Autodesk Inventor part; units mm, degrees
(part 2 of 2)
  line L320 (-28.6263, 16.0044) -> (-25.6449, 16.0044)
  line L321 (-25.6449, 18.3241) -> (-28.6263, 18.3241)
  line L322 (-29.7503, 19.4482) -> (-24.5209, 19.4482)
  line L323 (-29.5884, 13.8513) -> (-27.9357, 13.8513)
  line L324 (-29.5884, 12.8808) -> (-29.5884, 13.8513)
  line L325 (-29.7503, 14.8804) -> (-29.7503, 19.4482)
  line L326 (-26.6942, 13.8513) -> (-19.7097, 13.8513)
  line L327 (-23.8, 11.9101) -> (-23.8, 12.8808)
  line L328 (-25.8364, 11.9101) -> (-23.8, 11.9101)
  line L329 (-24.7124, 10.786) -> (-24.7124, 8.4664)
  line L330 (-21.731, 8.4664) -> (-21.731, 10.786)
  line L331 (-24.7124, 8.4664) -> (-21.731, 8.4664)
  line L332 (-21.731, 10.786) -> (-24.7124, 10.786)
  line L333 (-26.6942, 14.8804) -> (-26.6942, 13.8513)
  line L334 (-24.5209, 14.8804) -> (-26.6942, 14.8804)
  line L335 (-20.607, 11.9101) -> (-20.607, 7.3423)
  line L336 (-20.607, 7.3423) -> (-25.8364, 7.3423)
  line L337 (-25.8364, 7.3423) -> (-25.8364, 11.9101)
  line L338 (-27.9357, 14.8804) -> (-29.7503, 14.8804)
  line L339 (-45.1642, 41.8791) -> (-45.1642, 39.5595)
  line L340 (-49.1744, 38.4046) -> (-54.4039, 38.4046)
  line L341 (-53.2798, 39.5287) -> (-50.2985, 39.5287)
  line L342 (-50.2985, 39.5287) -> (-50.2985, 41.8484)
  line L343 (-47.0091, 45.0028) -> (-41.2208, 45.0028)
  line L344 (-51.0994, 42.9724) -> (-49.1744, 42.9724)
  line L345 (-50.2985, 41.8484) -> (-53.2798, 41.8484)
  line L346 (-55.1231, 45.0028) -> (-48.187, 45.0028)
  line L347 (-51.0994, 44.0323) -> (-51.0994, 42.9724)
  line L348 (-52.1825, 42.9724) -> (-52.1825, 44.0323)
  line L349 (-54.4039, 42.9724) -> (-52.1825, 42.9724)
  line L350 (-52.1825, 44.0323) -> (-55.1231, 44.0323)
  line L351 (-53.2798, 41.8484) -> (-53.2798, 39.5287)
  line L352 (-54.4039, 38.4046) -> (-54.4039, 42.9724)
  line L353 (-42.8734, 44.0323) -> (-42.8734, 43.0032)
  line L354 (-48.187, 45.0028) -> (-48.187, 45.9735)
  line L355 (-49.1744, 42.9724) -> (-49.1744, 38.4046)
  line L356 (-48.187, 45.9735) -> (-50.2022, 45.9735)
  line L357 (-55.1231, 44.0323) -> (-55.1231, 45.0028)
  line L358 (-46.2882, 38.4354) -> (-46.2882, 43.0032)
  line L359 (-42.1828, 39.5595) -> (-42.1828, 41.8791)
  line L360 (-42.1828, 41.8791) -> (-45.1642, 41.8791)
  line L361 (-45.1642, 39.5595) -> (-42.1828, 39.5595)
  line L362 (-41.0588, 38.4354) -> (-46.2882, 38.4354)
  line L363 (-41.2208, 44.0323) -> (-42.8734, 44.0323)
  line L364 (-41.2208, 45.0028) -> (-41.2208, 44.0323)
  line L365 (-41.0588, 43.0032) -> (-41.0588, 38.4354)
  line L366 (-44.1149, 44.0323) -> (-51.0994, 44.0323)
  line L367 (-47.0091, 45.9735) -> (-47.0091, 45.0028)
  line L368 (-44.9727, 45.9735) -> (-47.0091, 45.9735)
  line L369 (-46.0968, 47.0975) -> (-46.0968, 49.4172)
  line L370 (-49.0781, 49.4172) -> (-49.0781, 47.0975)
  line L371 (-46.0968, 49.4172) -> (-49.0781, 49.4172)
  line L372 (-49.0781, 47.0975) -> (-46.0968, 47.0975)
  line L373 (-44.1149, 43.0032) -> (-44.1149, 44.0323)
  line L374 (-46.2882, 43.0032) -> (-44.1149, 43.0032)
  line L375 (-50.2022, 45.9735) -> (-50.2022, 50.5413)
  line L376 (-50.2022, 50.5413) -> (-44.9727, 50.5413)
  line L377 (-44.9727, 50.5413) -> (-44.9727, 45.9735)
  line L378 (-42.8734, 43.0032) -> (-41.0588, 43.0032)
  line L379 (-29.0148, 57.3686) -> (-29.0148, 55.049)
  line L380 (-33.025, 53.8941) -> (-38.2545, 53.8941)
  line L381 (-37.1304, 55.0182) -> (-34.1491, 55.0182)
  line L382 (-34.1491, 55.0182) -> (-34.1491, 57.3379)
  line L383 (-30.8597, 60.4923) -> (-25.0713, 60.4923)
  line L384 (-34.95, 58.4619) -> (-33.025, 58.4619)
  line L385 (-34.1491, 57.3379) -> (-37.1304, 57.3379)
  line L386 (-38.9737, 60.4923) -> (-32.0376, 60.4923)
  line L387 (-34.95, 59.5218) -> (-34.95, 58.4619)
  line L388 (-36.0331, 58.4619) -> (-36.0331, 59.5218)
  line L389 (-38.2545, 58.4619) -> (-36.0331, 58.4619)
  line L390 (-36.0331, 59.5218) -> (-38.9737, 59.5218)
  line L391 (-37.1304, 57.3379) -> (-37.1304, 55.0182)
  line L392 (-38.2545, 53.8941) -> (-38.2545, 58.4619)
  line L393 (-26.724, 59.5218) -> (-26.724, 58.4927)
  line L394 (-32.0376, 60.4923) -> (-32.0376, 61.463)
  line L395 (-33.025, 58.4619) -> (-33.025, 53.8941)
  line L396 (-32.0376, 61.463) -> (-34.0527, 61.463)
  line L397 (-38.9737, 59.5218) -> (-38.9737, 60.4923)
  line L398 (-30.1388, 53.9249) -> (-30.1388, 58.4927)
  line L399 (-26.0334, 55.049) -> (-26.0334, 57.3686)
  line L400 (-26.0334, 57.3686) -> (-29.0148, 57.3686)
  line L401 (-29.0148, 55.049) -> (-26.0334, 55.049)
  line L402 (-24.9094, 53.9249) -> (-30.1388, 53.9249)
  line L403 (-25.0713, 59.5218) -> (-26.724, 59.5218)
  line L404 (-25.0713, 60.4923) -> (-25.0713, 59.5218)
  line L405 (-24.9094, 58.4927) -> (-24.9094, 53.9249)
  line L406 (-27.9655, 59.5218) -> (-34.95, 59.5218)
  line L407 (-30.8597, 61.463) -> (-30.8597, 60.4923)
  line L408 (-28.8233, 61.463) -> (-30.8597, 61.463)
  line L409 (-29.9473, 62.587) -> (-29.9473, 64.9067)
  line L410 (-32.9287, 64.9067) -> (-32.9287, 62.587)
  line L411 (-29.9473, 64.9067) -> (-32.9287, 64.9067)
  line L412 (-32.9287, 62.587) -> (-29.9473, 62.587)
  line L413 (-27.9655, 58.4927) -> (-27.9655, 59.5218)
  line L414 (-30.1388, 58.4927) -> (-27.9655, 58.4927)
  line L415 (-34.0527, 61.463) -> (-34.0527, 66.0308)
  line L416 (-34.0527, 66.0308) -> (-28.8233, 66.0308)
  line L417 (-28.8233, 66.0308) -> (-28.8233, 61.463)
  line L418 (-26.724, 58.4927) -> (-24.9094, 58.4927)
  line L419 (-32.0432, 45.0028) -> (-32.0432, 45.9735)
  line L420 (-32.0432, 45.9735) -> (-34.0584, 45.9735)
  line L421 (-27.9712, 44.0323) -> (-34.9556, 44.0323)
  line L422 (-32.9344, 47.0975) -> (-29.953, 47.0975)
  line L423 (-28.829, 45.9735) -> (-30.8654, 45.9735)
  line L424 (-32.9344, 49.4172) -> (-32.9344, 47.0975)
  line L425 (-34.0584, 45.9735) -> (-34.0584, 50.5413)
  line L426 (-29.953, 47.0975) -> (-29.953, 49.4172)
  line L427 (-29.953, 49.4172) -> (-32.9344, 49.4172)
  line L428 (-34.0584, 50.5413) -> (-28.829, 50.5413)
  line L429 (-28.829, 50.5413) -> (-28.829, 45.9735)
  line L430 (-30.8654, 45.9735) -> (-30.8654, 45.0028)
  line L431 (-33.0307, 38.4046) -> (-38.2601, 38.4046)
  line L432 (-37.1361, 39.5287) -> (-34.1547, 39.5287)
  line L433 (-34.1547, 39.5287) -> (-34.1547, 41.8484)
  line L434 (-34.9556, 42.9724) -> (-33.0307, 42.9724)
  line L435 (-34.1547, 41.8484) -> (-37.1361, 41.8484)
  line L436 (-38.9793, 45.0028) -> (-32.0432, 45.0028)
  line L437 (-36.0387, 42.9724) -> (-36.0387, 44.0323)
  line L438 (-38.9793, 44.0323) -> (-38.9793, 45.0028)
  line L439 (-36.0387, 44.0323) -> (-38.9793, 44.0323)
  line L440 (-38.2601, 42.9724) -> (-36.0387, 42.9724)
  line L441 (-37.1361, 41.8484) -> (-37.1361, 39.5287)
  line L442 (-38.2601, 38.4046) -> (-38.2601, 42.9724)
  line L443 (-34.9556, 44.0323) -> (-34.9556, 42.9724)
  line L444 (-29.0204, 41.8791) -> (-29.0204, 39.5595)
  line L445 (-30.8654, 45.0028) -> (-25.077, 45.0028)
  line L446 (-26.7296, 44.0323) -> (-26.7296, 43.0032)
  line L447 (-33.0307, 42.9724) -> (-33.0307, 38.4046)
  line L448 (-30.1445, 38.4354) -> (-30.1445, 43.0032)
  line L449 (-30.1445, 43.0032) -> (-27.9712, 43.0032)
  line L450 (-27.9712, 43.0032) -> (-27.9712, 44.0323)
  line L451 (-25.077, 45.0028) -> (-25.077, 44.0323)
  line L452 (-25.077, 44.0323) -> (-26.7296, 44.0323)
  line L453 (-26.0391, 41.8791) -> (-29.0204, 41.8791)
  line L454 (-26.7296, 43.0032) -> (-24.915, 43.0032)
  line L455 (-29.0204, 39.5595) -> (-26.0391, 39.5595)
  line L456 (-24.915, 38.4354) -> (-30.1445, 38.4354)
  line L457 (-24.915, 43.0032) -> (-24.915, 38.4354)
  line L458 (-26.0391, 39.5595) -> (-26.0391, 41.8791)
  line L459 (-15.8995, 45.0028) -> (-15.8995, 45.9735)
  line L460 (-15.8995, 45.9735) -> (-17.9146, 45.9735)
  line L461 (-11.8274, 44.0323) -> (-18.8118, 44.0323)
  line L462 (-16.7906, 47.0975) -> (-13.8092, 47.0975)
  line L463 (-12.6852, 45.9735) -> (-14.7216, 45.9735)
  line L464 (-16.7906, 49.4172) -> (-16.7906, 47.0975)
  line L465 (-17.9146, 45.9735) -> (-17.9146, 50.5413)
  line L466 (-13.8092, 47.0975) -> (-13.8092, 49.4172)
  line L467 (-13.8092, 49.4172) -> (-16.7906, 49.4172)
  line L468 (-17.9146, 50.5413) -> (-12.6852, 50.5413)
  line L469 (-12.6852, 50.5413) -> (-12.6852, 45.9735)
  line L470 (-14.7216, 45.9735) -> (-14.7216, 45.0028)
  line L471 (-16.8869, 38.4046) -> (-22.1163, 38.4046)
  line L472 (-20.9923, 39.5287) -> (-18.0109, 39.5287)
  line L473 (-18.0109, 39.5287) -> (-18.0109, 41.8484)
  line L474 (-18.8118, 42.9724) -> (-16.8869, 42.9724)
  line L475 (-18.0109, 41.8484) -> (-20.9923, 41.8484)
  line L476 (-22.8356, 45.0028) -> (-15.8995, 45.0028)
  line L477 (-19.895, 42.9724) -> (-19.895, 44.0323)
  line L478 (-22.8356, 44.0323) -> (-22.8356, 45.0028)
  line L479 (-19.895, 44.0323) -> (-22.8356, 44.0323)
  line L480 (-22.1163, 42.9724) -> (-19.895, 42.9724)
  line L481 (-20.9923, 41.8484) -> (-20.9923, 39.5287)
  line L482 (-22.1163, 38.4046) -> (-22.1163, 42.9724)
  line L483 (-18.8118, 44.0323) -> (-18.8118, 42.9724)
  line L484 (-12.8767, 41.8791) -> (-12.8767, 39.5595)
  line L485 (-14.7216, 45.0028) -> (-8.9332, 45.0028)
  line L486 (-10.5859, 44.0323) -> (-10.5859, 43.0032)
  line L487 (-16.8869, 42.9724) -> (-16.8869, 38.4046)
  line L488 (-14.0007, 38.4354) -> (-14.0007, 43.0032)
  line L489 (-14.0007, 43.0032) -> (-11.8274, 43.0032)
  line L490 (-11.8274, 43.0032) -> (-11.8274, 44.0323)
  line L491 (-8.9332, 45.0028) -> (-8.9332, 44.0323)
  line L492 (-8.9332, 44.0323) -> (-10.5859, 44.0323)
  line L493 (-9.8953, 41.8791) -> (-12.8767, 41.8791)
  line L494 (-10.5859, 43.0032) -> (-8.7712, 43.0032)
  line L495 (-12.8767, 39.5595) -> (-9.8953, 39.5595)
  line L496 (-8.7712, 38.4354) -> (-14.0007, 38.4354)
  line L497 (-8.7712, 43.0032) -> (-8.7712, 38.4354)
  line L498 (-9.8953, 39.5595) -> (-9.8953, 41.8791)
  spline S0 degree 2 poles (-57.0967, 82.1505) (-57.0967, 82.9326) (-56.5863, 84.2335) (-56.1417, 84.7028) knots 0 0 0 1 2 2 2
  spline S1 degree 2 poles (-56.1417, 84.7028) (-55.7218, 85.1557) (-54.495, 85.6579) (-53.8692, 85.6579) knots 0 0 0 1 2 2 2
  spline S2 degree 2 poles (-53.8692, 85.6579) (-53.1694, 85.6579) (-52.0332, 85.1886) (-51.6133, 84.744) knots 0 0 0 1 2 2 2
  spline S3 degree 2 poles (-51.6133, 84.744) (-51.0864, 84.1841) (-50.51, 82.3728) (-50.51, 80.9813) knots 0 0 0 1 2 2 2
  spline S4 degree 2 poles (-50.51, 80.9813) (-50.51, 79.7216) (-51.0781, 77.4657) (-51.6298, 76.7164) knots 0 0 0 1 2 2 2
  spline S5 degree 2 poles (-51.6298, 76.7164) (-52.2143, 75.926) (-53.861, 75.0945) (-55.0631, 75.0945) knots 0 0 0 1 2 2 2
  spline S6 degree 2 poles (-55.0631, 75.0945) (-55.3348, 75.0945) (-55.9523, 75.1521) (-56.2158, 75.2344) knots 0 0 0 1 2 2 2
  line L499 (-56.2158, 75.2344) -> (-56.2158, 76.5435)
  line L500 (-56.2158, 76.5435) -> (-56.1499, 76.5435)
  spline S7 degree 2 poles (-56.1499, 76.5435) (-55.977, 76.4447) (-55.2525, 76.2718) (-54.882, 76.2718) knots 0 0 0 1 2 2 2
  spline S8 degree 2 poles (-54.882, 76.2718) (-53.5481, 76.2718) (-52.025, 78.0338) (-51.9179, 79.664) knots 0 0 0 1 2 2 2
  spline S9 degree 2 poles (-51.9179, 79.664) (-52.4613, 79.2935) (-53.4493, 78.9559) (-54.0339, 78.9559) knots 0 0 0 1 2 2 2
  spline S10 degree 2 poles (-54.0339, 78.9559) (-54.5938, 78.9559) (-55.5242, 79.2029) (-55.9935, 79.557) knots 0 0 0 1 2 2 2
  spline S11 degree 2 poles (-55.9935, 79.557) (-56.5369, 79.9769) (-57.0967, 81.253) (-57.0967, 82.1505) knots 0 0 0 1 2 2 2
  spline S12 degree 2 poles (-51.885, 81.286) (-51.885, 82.3151) (-52.2637, 83.616) (-52.6013, 83.97) knots 0 0 0 1 2 2 2
  spline S13 degree 2 poles (-52.6013, 83.97) (-52.8977, 84.2994) (-53.5152, 84.5464) (-53.8775, 84.5464) knots 0 0 0 1 2 2 2
  spline S14 degree 2 poles (-53.8775, 84.5464) (-54.7173, 84.5464) (-55.7135, 83.3443) (-55.7135, 82.2081) knots 0 0 0 1 2 2 2
  spline S15 degree 2 poles (-55.7135, 82.2081) (-55.7135, 81.5659) (-55.3842, 80.7343) (-55.0219, 80.4379) knots 0 0 0 1 2 2 2
  spline S16 degree 2 poles (-55.0219, 80.4379) (-54.7585, 80.2239) (-54.108, 80.0839) (-53.7293, 80.0839) knots 0 0 0 1 2 2 2
  spline S17 degree 2 poles (-53.7293, 80.0839) (-53.2929, 80.0839) (-52.2884, 80.3885) (-51.9097, 80.6438) knots 0 0 0 1 2 2 2
  spline S18 degree 2 poles (-51.9097, 80.6438) (-51.9015, 80.7426) (-51.885, 81.0801) (-51.885, 81.286) knots 0 0 0 1 2 2 2
  spline S19 degree 2 poles (-6.4033, 6.9192) (-6.4033, 6.137) (-6.9137, 4.8361) (-7.3583, 4.3668) knots 0 0 0 1 2 2 2
  spline S20 degree 2 poles (-7.3583, 4.3668) (-7.7782, 3.914) (-9.005, 3.4117) (-9.6308, 3.4117) knots 0 0 0 1 2 2 2
  spline S21 degree 2 poles (-9.6308, 3.4117) (-10.3306, 3.4117) (-11.4668, 3.881) (-11.8867, 4.3257) knots 0 0 0 1 2 2 2
  spline S22 degree 2 poles (-11.8867, 4.3257) (-12.4136, 4.8855) (-12.99, 6.6969) (-12.99, 8.0883) knots 0 0 0 1 2 2 2
  spline S23 degree 2 poles (-12.99, 8.0883) (-12.99, 9.348) (-12.4219, 11.604) (-11.8702, 12.3532) knots 0 0 0 1 2 2 2
  spline S24 degree 2 poles (-11.8702, 12.3532) (-11.2857, 13.1436) (-9.639, 13.9752) (-8.4369, 13.9752) knots 0 0 0 1 2 2 2
  spline S25 degree 2 poles (-8.4369, 13.9752) (-8.1652, 13.9752) (-7.5477, 13.9175) (-7.2842, 13.8352) knots 0 0 0 1 2 2 2
  line L501 (-7.2842, 13.8352) -> (-7.2842, 12.5261)
  line L502 (-7.2842, 12.5261) -> (-7.3501, 12.5261)
  spline S26 degree 2 poles (-7.3501, 12.5261) (-7.523, 12.6249) (-8.2475, 12.7978) (-8.618, 12.7978) knots 0 0 0 1 2 2 2
  spline S27 degree 2 poles (-8.618, 12.7978) (-9.9519, 12.7978) (-11.475, 11.0359) (-11.5821, 9.4057) knots 0 0 0 1 2 2 2
  spline S28 degree 2 poles (-11.5821, 9.4057) (-11.0387, 9.7762) (-10.0507, 10.1137) (-9.4661, 10.1137) knots 0 0 0 1 2 2 2
  spline S29 degree 2 poles (-9.4661, 10.1137) (-8.9062, 10.1137) (-7.9758, 9.8667) (-7.5065, 9.5127) knots 0 0 0 1 2 2 2
  spline S30 degree 2 poles (-7.5065, 9.5127) (-6.9631, 9.0928) (-6.4033, 7.8166) (-6.4033, 6.9192) knots 0 0 0 1 2 2 2
  spline S31 degree 2 poles (-11.615, 7.7837) (-11.615, 6.7545) (-11.2363, 5.4536) (-10.8987, 5.0996) knots 0 0 0 1 2 2 2
  spline S32 degree 2 poles (-10.8987, 5.0996) (-10.6023, 4.7703) (-9.9848, 4.5233) (-9.6225, 4.5233) knots 0 0 0 1 2 2 2
  spline S33 degree 2 poles (-9.6225, 4.5233) (-8.7827, 4.5233) (-7.7865, 5.7253) (-7.7865, 6.8615) knots 0 0 0 1 2 2 2
  spline S34 degree 2 poles (-7.7865, 6.8615) (-7.7865, 7.5037) (-8.1158, 8.3353) (-8.4781, 8.6317) knots 0 0 0 1 2 2 2
  spline S35 degree 2 poles (-8.4781, 8.6317) (-8.7415, 8.8458) (-9.392, 8.9857) (-9.7707, 8.9857) knots 0 0 0 1 2 2 2
  spline S36 degree 2 poles (-9.7707, 8.9857) (-10.2071, 8.9857) (-11.2116, 8.6811) (-11.5903, 8.4259) knots 0 0 0 1 2 2 2
  spline S37 degree 2 poles (-11.5903, 8.4259) (-11.5985, 8.3271) (-11.615, 7.9895) (-11.615, 7.7837) knots 0 0 0 1 2 2 2
  spline S38 degree 2 poles (-6.4033, 6.9192) (-6.4033, 6.137) (-6.9137, 4.8361) (-7.3583, 4.3668) knots 0 0 0 1 2 2 2
  spline S39 degree 2 poles (-7.3583, 4.3668) (-7.7782, 3.914) (-9.005, 3.4117) (-9.6308, 3.4117) knots 0 0 0 1 2 2 2
  spline S40 degree 2 poles (-9.6308, 3.4117) (-10.3306, 3.4117) (-11.4668, 3.881) (-11.8867, 4.3257) knots 0 0 0 1 2 2 2
  spline S41 degree 2 poles (-11.8867, 4.3257) (-12.4136, 4.8855) (-12.99, 6.6969) (-12.99, 8.0883) knots 0 0 0 1 2 2 2
  spline S42 degree 2 poles (-12.99, 8.0883) (-12.99, 9.348) (-12.4219, 11.604) (-11.8702, 12.3532) knots 0 0 0 1 2 2 2
  spline S43 degree 2 poles (-11.8702, 12.3532) (-11.2857, 13.1436) (-9.639, 13.9752) (-8.4369, 13.9752) knots 0 0 0 1 2 2 2
  spline S44 degree 2 poles (-8.4369, 13.9752) (-8.1652, 13.9752) (-7.5477, 13.9175) (-7.2842, 13.8352) knots 0 0 0 1 2 2 2
  line L503 (-7.2842, 13.8352) -> (-7.2842, 12.5261)
  line L504 (-7.2842, 12.5261) -> (-7.3501, 12.5261)
  spline S45 degree 2 poles (-7.3501, 12.5261) (-7.523, 12.6249) (-8.2475, 12.7978) (-8.618, 12.7978) knots 0 0 0 1 2 2 2
  spline S46 degree 2 poles (-8.618, 12.7978) (-9.9519, 12.7978) (-11.475, 11.0359) (-11.5821, 9.4057) knots 0 0 0 1 2 2 2
  spline S47 degree 2 poles (-11.5821, 9.4057) (-11.0387, 9.7762) (-10.0507, 10.1137) (-9.4661, 10.1137) knots 0 0 0 1 2 2 2
  spline S48 degree 2 poles (-9.4661, 10.1137) (-8.9062, 10.1137) (-7.9758, 9.8667) (-7.5065, 9.5127) knots 0 0 0 1 2 2 2
  spline S49 degree 2 poles (-7.5065, 9.5127) (-6.9631, 9.0928) (-6.4033, 7.8166) (-6.4033, 6.9192) knots 0 0 0 1 2 2 2
  spline S50 degree 2 poles (-11.615, 7.7837) (-11.615, 6.7545) (-11.2363, 5.4536) (-10.8987, 5.0996) knots 0 0 0 1 2 2 2
  spline S51 degree 2 poles (-10.8987, 5.0996) (-10.6023, 4.7703) (-9.9848, 4.5233) (-9.6225, 4.5233) knots 0 0 0 1 2 2 2
  spline S52 degree 2 poles (-9.6225, 4.5233) (-8.7827, 4.5233) (-7.7865, 5.7253) (-7.7865, 6.8615) knots 0 0 0 1 2 2 2
  spline S53 degree 2 poles (-7.7865, 6.8615) (-7.7865, 7.5037) (-8.1158, 8.3353) (-8.4781, 8.6317) knots 0 0 0 1 2 2 2
  spline S54 degree 2 poles (-8.4781, 8.6317) (-8.7415, 8.8458) (-9.392, 8.9857) (-9.7707, 8.9857) knots 0 0 0 1 2 2 2
  spline S55 degree 2 poles (-9.7707, 8.9857) (-10.2071, 8.9857) (-11.2116, 8.6811) (-11.5903, 8.4259) knots 0 0 0 1 2 2 2
  spline S56 degree 2 poles (-11.5903, 8.4259) (-11.5985, 8.3271) (-11.615, 7.9895) (-11.615, 7.7837) knots 0 0 0 1 2 2 2
  spline S57 degree 2 poles (-57.0967, 82.1505) (-57.0967, 82.9326) (-56.5863, 84.2335) (-56.1417, 84.7028) knots 0 0 0 1 2 2 2
  spline S58 degree 2 poles (-56.1417, 84.7028) (-55.7218, 85.1557) (-54.495, 85.6579) (-53.8692, 85.6579) knots 0 0 0 1 2 2 2
  spline S59 degree 2 poles (-53.8692, 85.6579) (-53.1694, 85.6579) (-52.0332, 85.1886) (-51.6133, 84.744) knots 0 0 0 1 2 2 2
  spline S60 degree 2 poles (-51.6133, 84.744) (-51.0864, 84.1841) (-50.51, 82.3728) (-50.51, 80.9813) knots 0 0 0 1 2 2 2
  spline S61 degree 2 poles (-50.51, 80.9813) (-50.51, 79.7216) (-51.0781, 77.4657) (-51.6298, 76.7164) knots 0 0 0 1 2 2 2
  spline S62 degree 2 poles (-51.6298, 76.7164) (-52.2143, 75.926) (-53.861, 75.0945) (-55.0631, 75.0945) knots 0 0 0 1 2 2 2
  spline S63 degree 2 poles (-55.0631, 75.0945) (-55.3348, 75.0945) (-55.9523, 75.1521) (-56.2158, 75.2344) knots 0 0 0 1 2 2 2
  line L505 (-56.2158, 75.2344) -> (-56.2158, 76.5435)
  line L506 (-56.2158, 76.5435) -> (-56.1499, 76.5435)
  spline S64 degree 2 poles (-56.1499, 76.5435) (-55.977, 76.4447) (-55.2525, 76.2718) (-54.882, 76.2718) knots 0 0 0 1 2 2 2
  spline S65 degree 2 poles (-54.882, 76.2718) (-53.5481, 76.2718) (-52.025, 78.0338) (-51.9179, 79.664) knots 0 0 0 1 2 2 2
  spline S66 degree 2 poles (-51.9179, 79.664) (-52.4613, 79.2935) (-53.4493, 78.9559) (-54.0339, 78.9559) knots 0 0 0 1 2 2 2
  spline S67 degree 2 poles (-54.0339, 78.9559) (-54.5938, 78.9559) (-55.5242, 79.2029) (-55.9935, 79.557) knots 0 0 0 1 2 2 2
  spline S68 degree 2 poles (-55.9935, 79.557) (-56.5369, 79.9769) (-57.0967, 81.253) (-57.0967, 82.1505) knots 0 0 0 1 2 2 2
  spline S69 degree 2 poles (-51.885, 81.286) (-51.885, 82.3151) (-52.2637, 83.616) (-52.6013, 83.97) knots 0 0 0 1 2 2 2
  spline S70 degree 2 poles (-52.6013, 83.97) (-52.8977, 84.2994) (-53.5152, 84.5464) (-53.8775, 84.5464) knots 0 0 0 1 2 2 2
  spline S71 degree 2 poles (-53.8775, 84.5464) (-54.7173, 84.5464) (-55.7135, 83.3443) (-55.7135, 82.2081) knots 0 0 0 1 2 2 2
  spline S72 degree 2 poles (-55.7135, 82.2081) (-55.7135, 81.5659) (-55.3842, 80.7343) (-55.0219, 80.4379) knots 0 0 0 1 2 2 2
  spline S73 degree 2 poles (-55.0219, 80.4379) (-54.7585, 80.2239) (-54.108, 80.0839) (-53.7293, 80.0839) knots 0 0 0 1 2 2 2
  spline S74 degree 2 poles (-53.7293, 80.0839) (-53.2929, 80.0839) (-52.2884, 80.3885) (-51.9097, 80.6438) knots 0 0 0 1 2 2 2
  spline S75 degree 2 poles (-51.9097, 80.6438) (-51.9015, 80.7426) (-51.885, 81.0801) (-51.885, 81.286) knots 0 0 0 1 2 2 2
  point P0 (-40.5846, 75.534)
  point P1 (-53.7479, 68.8958)
  point P2 (-9.7521, 20.0042)
  point P3 (-41.8348, 101.4209)
  point P4 (-40.5846, 75.534)
  point P5 (-53.7479, 68.8958)
  point P6 (-9.7521, 20.0042)
  point P7 (-1, 6.9835)
  point P8 (-22.9154, 75.534)
  point P9 (-31.7444, 28.893)
  point P10 (-31.7444, 28.893)
  point P11 (-22.9154, 75.534)
  point P12 (-22.9154, 75.534)
  point P13 (-40.5846, 13.366)
  point P14 (-22.9154, 13.366)
  point P15 (-40.5846, 13.366)
  point P16 (-40.5846, 13.366)
  point P17 (-22.9154, 13.366)
  point P18 (-22.9154, 13.366)
  point P19 (-47.8938, 44.5175)
  point P20 (-47.8938, 44.5175)
  point P21 (-31.7444, 60.007)
  point P22 (-31.7444, 60.007)
  point P23 (-31.7444, 60.007)
  point P24 (-31.7444, 28.893)
  point P25 (-31.75, 44.45)
  point P26 (-15.6062, 44.5175)
  point P27 (-31.75, 44.5175)
  point P28 (-31.75, 44.5175)
  point P29 (-15.6062, 44.5175)
  point P30 (-15.6062, 44.5175)
  dimension "d155" = 8.4153
  dimension "d157" = 0.508
  dimension "d158" = 4.5466
  dimension "d159" = 0.508
  dimension "d160" = 4.5466
  constraints: 972 end point, 50 parallel, 20 perpendicular, 14 horizontal, 6 midpoint, 3 symmetric about line, 14 other
  measures "d155" distance of L174.end L172.start
  measures "d157" distance between parallel lines of L7 L173
  measures "d158" distance from line of point (-1, 6.983) L172
  measures "d159" distance between parallel lines of L6 L168
  measures "d160" distance between parallel lines of L4 L171
extrude "Extrusion20" add sketch "Sketch17" along normal blind 0.4 contours L48 L49 L73 L71 L76 L69 L86 L79 L85 L67 L62 L68 L84 L80 L87 L77 L82 L60 L55 L61 L81 L78 L83 L70 L75 L72 L74 L50 | L88 L89 L113 L111 L116 L109 L126 L119 L125 L107 L102 L108 L124 L120 L127 L117 L122 L100 L95 L101 L121 L118 L123 L110 L115 L112 L114 L90 | L128 L129 L153 L151 L156 L149 L166 L159 L165 L147 L142 L148 L164 L160 L167 L157 L162 L140 L135 L141 L161 L158 L163 L150 L155 L152 L154 L130 | L179 L185 L186 L189 L190 L191 L194 L192 L193 L209 L207 L208 L217 L216 L197 L198 L199 L195 L206 L205 L204 L201 L215 L214 L218 L188 L183 L184 | L219 L225 L226 L229 L230 L231 L234 L232 L233 L249 L247 L248 L257 L256 L237 L238 L239 L235 L246 L245 L244 L241 L255 L254 L258 L228 L223 L224 | L260 L272 L269 L268 L270 L277 L266 L274 L276 L295 L296 L297 L288 L287 L263 L284 L283 L273 L298 L285 L282 L278 L294 L293 L286 L267 L264 L275 | L300 L312 L309 L308 L310 L317 L306 L314 L316 L335 L336 L337 L328 L327 L303 L324 L323 L313 L338 L325 L322 L318 L334 L333 L326 L307 L304 L315 | L340 L352 L349 L348 L350 L357 L346 L354 L356 L375 L376 L377 L368 L367 L343 L364 L363 L353 L378 L365 L362 L358 L374 L373 L366 L347 L344 L355 | L380 L392 L389 L388 L390 L397 L386 L394 L396 L415 L416 L417 L408 L407 L383 L404 L403 L393 L418 L405 L402 L398 L414 L413 L406 L387 L384 L395 | L419 L420 L425 L428 L429 L423 L430 L445 L451 L452 L446 L454 L457 L456 L448 L449 L450 L421 L443 L434 L447 L431 L442 L440 L437 L439 L438 L436 | L459 L460 L465 L468 L469 L463 L470 L485 L491 L492 L486 L494 L497 L496 L488 L489 L490 L461 L483 L474 L487 L471 L482 L480 L477 L479 L478 L476 | S0 S1 S2 S3 S4 S5 S6 L499 L500 S7 S8 S9 S10 S11 | S19 S20 S21 S22 S23 S24 S25 L501 L502 S26 S27 S28 S29 S30 bodies 2
sketch "Sketch18" plane through (0, 0, -0.2) normal (0, 0, -1) x (-1, 0, 0)
  line L0 (0, 0) -> (-63.5, 0)
  line L1 (-63.5, 0) -> (-63.5, 88.9)
  line L2 (-63.5, 88.9) -> (0, 88.9)
  line L3 (0, 88.9) -> (0, 0)
  constraints: 8 end point, 2 parallel, 1 horizontal, 1 perpendicular
extrude "Extrusion21" add sketch "Sketch18" along normal blind 0.4 bodies 3
fillet "Fillet2" radius 3.175 8 edges at (63.5, 0, 0.2) (63.5, 88.9, 0.2) (0, 0, 0.2) (0, 88.9, 0.2) (63.5, 0, -0.3) (63.5, 88.9, -0.3) (0, 0, -0.3) (0, 88.9, -0.3)
extrude "Extrusion22" cut sketch "Sketch17" along normal blind 0.4 contours L48 L49 L73 L71 L76 L69 L86 L79 L85 L67 L62 L68 L84 L80 L87 L77 L82 L60 L55 L61 L81 L78 L83 L70 L75 L72 L74 L50 | L88 L89 L113 L111 L116 L109 L126 L119 L125 L107 L102 L108 L124 L120 L127 L117 L122 L100 L95 L101 L121 L118 L123 L110 L115 L112 L114 L90 | L128 L129 L153 L151 L156 L149 L166 L159 L165 L147 L142 L148 L164 L160 L167 L157 L162 L140 L135 L141 L161 L158 L163 L150 L155 L152 L154 L130 | L179 L185 L186 L189 L190 L191 L194 L192 L193 L209 L207 L208 L217 L216 L197 L198 L199 L195 L206 L205 L204 L201 L215 L214 L218 L188 L183 L184 | L219 L225 L226 L229 L230 L231 L234 L232 L233 L249 L247 L248 L257 L256 L237 L238 L239 L235 L246 L245 L244 L241 L255 L254 L258 L228 L223 L224 | L260 L272 L269 L268 L270 L277 L266 L274 L276 L295 L296 L297 L288 L287 L263 L284 L283 L273 L298 L285 L282 L278 L294 L293 L286 L267 L264 L275 | L300 L312 L309 L308 L310 L317 L306 L314 L316 L335 L336 L337 L328 L327 L303 L324 L323 L313 L338 L325 L322 L318 L334 L333 L326 L307 L304 L315 | L340 L352 L349 L348 L350 L357 L346 L354 L356 L375 L376 L377 L368 L367 L343 L364 L363 L353 L378 L365 L362 L358 L374 L373 L366 L347 L344 L355 | L380 L392 L389 L388 L390 L397 L386 L394 L396 L415 L416 L417 L408 L407 L383 L404 L403 L393 L418 L405 L402 L398 L414 L413 L406 L387 L384 L395 | L419 L420 L425 L428 L429 L423 L430 L445 L451 L452 L446 L454 L457 L456 L448 L449 L450 L421 L443 L434 L447 L431 L442 L440 L437 L439 L438 L436 | L459 L460 L465 L468 L469 L463 L470 L485 L491 L492 L486 L494 L497 L496 L488 L489 L490 L461 L483 L474 L487 L471 L482 L480 L477 L479 L478 L476 | S0 S1 S2 S3 S4 S5 S6 L499 L500 S7 S8 S9 S10 S11 | S19 S20 S21 S22 S23 S24 S25 L501 L502 S26 S27 S28 S29 S30 bodies 3
